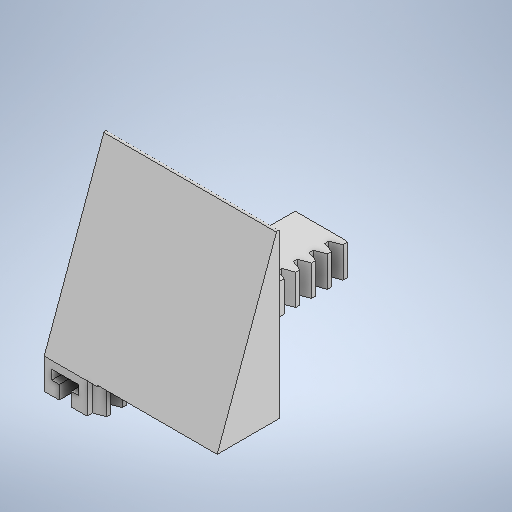
# Autodesk Inventor part: sg90 claw finger
Saved by Autodesk Inventor 2025 (Build 290162000, 162)
## iProperties
Created: 2025-05-11
Part Number: sg90 claw finger
Material: 一般
Document SubType Name: Modeling
Designer: gavin
Density: 1 g/cm^3
Appearance: 預設
Author: gavin
## iProperties of the stored document sg90 claw finger_3D 列印.ipt
Created: 2025-05-11
Part Number: sg90 claw finger_3D 列印
Material: 一般
Document SubType Name: Modeling
Designer: gavin
Density: 1 g/cm^3
Appearance: 預設
Author: gavin
Autodesk Inventor part; units mm, degrees
ref_plane "YZ Plane" through (0, 0, 0) normal (1, 0, 0) x (0, 1, 0)
ref_plane "XZ Plane" through (0, 0, 0) normal (0, 1, 0) x (-1, 0, 0)
sketch "草圖1" plane through (0, 0, 0) normal (0, 0, 1) x (1, 0, 0)
  line L0 (0, -4.2926) -> (-28, -4.2926) projected
  line L1 (0, -4.2926) -> (0, 6.9129) projected
  line L2 (0, 6.9129) -> (1.5, 6.9129) projected
  line L3 (1.5, 6.9129) -> (1.5, 8.4129) projected
  line L4 (1.5, 8.4129) -> (-3.5, 8.4129) projected
  line L5 (-3.5, 8.4129) -> (-3.5, 6.9129) projected
  line L6 (-3.5, 6.9129) -> (-2, 6.9129) projected
  line L7 (-2, 6.9129) -> (-2, 3.81) projected
  line L8 (-2, 3.81) -> (-26, 3.81) projected
  line L9 (-26, 3.81) -> (-26, 6.9129) projected
  line L10 (-26, 6.9129) -> (-24.5, 6.9129) projected
  line L11 (-24.5, 6.9129) -> (-24.5, 8.4129) projected
  line L12 (-24.5, 8.4129) -> (-29.5, 8.4129) projected
  line L13 (-29.5, 8.4129) -> (-29.5, 6.9129) projected
  line L14 (-29.5, 6.9129) -> (-28, 6.9129) projected
  line L15 (-28, -4.2926) -> (-28, 6.9129) projected
  line L16 (-25.8, 4.01) -> (-2.2, 4.01)
  line L17 (-2.2, 4.01) -> (-2.2, 6.7129)
  line L18 (-2.2, 6.7129) -> (-3.7, 6.7129)
  line L19 (-3.7, 6.7129) -> (-3.7, 8.6129)
  line L20 (-3.7, 8.6129) -> (1.7, 8.6129)
  line L21 (1.7, 8.6129) -> (1.7, 6.7129)
  line L22 (1.7, 6.7129) -> (0.2, 6.7129)
  line L23 (0.2, 6.7129) -> (0.2, -4.4926)
  line L24 (0.2, -4.4926) -> (-28.2, -4.4926)
  line L25 (-28.2, -4.4926) -> (-28.2, 6.7129)
  line L26 (-28.2, 6.7129) -> (-29.7, 6.7129)
  line L27 (-29.7, 6.7129) -> (-29.7, 8.6129)
  line L28 (-29.7, 8.6129) -> (-24.3, 8.6129)
  line L29 (-24.3, 8.6129) -> (-24.3, 6.7129)
  line L30 (-24.3, 6.7129) -> (-25.8, 6.7129)
  line L31 (-25.8, 6.7129) -> (-25.8, 4.01)
  line L32 (-23.8, 4.01) -> (-23.8, 10.1129)
  line L33 (-23.8, 10.1129) -> (-31.2, 10.1129)
  line L34 (-31.2, 10.1129) -> (-31.2, 4.01)
  line L35 (-31.2, 4.01) -> (-28.2, 4.01)
  point P0 (0, 0)
  point P1 (-31.2, 7.0615)
  point P2 (-23.8, 7.0615)
  point P3 (-29.7, 4.01)
  dimension "d0" = 0.2
  dimension "d1" = 1.5
  dimension "d2" = 0.5
  dimension "d3" = 1.5
  constraints: 40 end point, 3 midpoint, 3 perpendicular, 2 point on line, 1 horizontal alignment, 1 vertical, 15 other
  measures "d0" distance between parallel lines of L8 L16
  measures "d1" distance from line of point (-31.2, 7.061) L27
  measures "d2" distance from line of point (-23.8, 7.061) L29
  measures "d3" distance between parallel lines of L28 L33
ref_plane "工作平面1" through (-29.5, -4.2926, -50) normal (0, 0, -1) x (0, 1, 0)
extrude "擠出1" add sketch "草圖1" against normal up to surface (50 mm away) contours L31 L30 L29 L28 L27 L26 L25 L35 L34 L33 L32 L16
sketch "草圖2" plane through (-31.2, 10.1129, 0) normal (0, 1, 0) x (1, 0, 0)
  circle A0 centre (17.2, 25) radius 1 projected
  spline S0 degree 3 poles (20.638, 31.1549) (20.6159, 31.1126) (20.5826, 31.049) (20.5316, 30.968) (20.489, 30.9103) (20.4434, 30.8548) (20.393, 30.8037) (20.3395, 30.7558) (20.281, 30.7141) (20.2184, 30.6788) (20.152, 30.6512) (20.0825, 30.6328) (20.011, 30.6244) (19.9391, 30.627) (19.8684, 30.6405) (19.8012, 30.6662) (19.7364, 30.6968) (19.6702, 30.7245) (19.6062, 30.7572) (19.5488, 30.8007) (19.4988, 30.8524) (19.4572, 30.9112) (19.4244, 30.9752) (19.4005, 31.043) (19.3848, 31.1131) (19.3766, 31.1845) (19.3764, 31.2563) (19.3807, 31.328) (19.3915, 31.3989) (19.4058, 31.4693) (19.4319, 31.5613) (19.4569, 31.6286) (19.4735, 31.6734) knots -0.22945 -0.22945 -0.22945 -0.22945 -0.21511 -0.207939 -0.200767 -0.193594 -0.186424 -0.179252 -0.17208 -0.164908 -0.157739 -0.150569 -0.143398 -0.136229 -0.129062 -0.121897 -0.114725 -0.107553 -0.100388 -0.093221 -0.086052 -0.078881 -0.071711 -0.064542 -0.05737 -0.050197 -0.043026 -0.035856 -0.028683 -0.021511 -0.01434 0 0 0 0 projected
  spline S1 degree 3 poles (19.4735, 31.6734) (19.4811, 31.7051) (19.4963, 31.7685) (19.5071, 31.8658) (19.5135, 31.9634) (19.5154, 32.0938) (19.5078, 32.2567) (19.4855, 32.451) (19.4519, 32.6437) (19.4081, 32.8343) (19.3559, 33.0228) (19.3139, 33.1463) (19.293, 33.208) knots -0.156401 -0.156401 -0.156401 -0.156401 -0.146631 -0.136856 -0.127081 -0.117305 -0.097756 -0.078206 -0.058655 -0.039103 -0.019552 0 0 0 0 projected
  arc A1 (19.293, 33.208) -> (18.6265, 33.3497) centre (17.2, 25) ccw projected
  spline S2 degree 3 poles (18.6265, 33.3497) (18.5822, 33.3018) (18.4937, 33.2061) (18.3693, 33.0552) (18.2517, 32.8988) (18.1427, 32.7364) (18.0433, 32.568) (17.9701, 32.4222) (17.9188, 32.3023) (17.8849, 32.2106) (17.8553, 32.1173) (17.8433, 32.0532) (17.8374, 32.0212) knots -0.156401 -0.156401 -0.156401 -0.156401 -0.13685 -0.117298 -0.097746 -0.078195 -0.058645 -0.039096 -0.02932 -0.019545 -0.00977 0 0 0 0 projected
  spline S3 degree 3 poles (17.8374, 32.0212) (17.8343, 31.9735) (17.8298, 31.9019) (17.8162, 31.8071) (17.8007, 31.7371) (17.7816, 31.6679) (17.7564, 31.6007) (17.727, 31.5352) (17.6905, 31.4733) (17.6477, 31.4156) (17.5983, 31.3633) (17.5422, 31.3182) (17.4804, 31.2814) (17.4136, 31.2546) (17.3435, 31.2382) (17.2717, 31.2343) (17.2, 31.2359) (17.1283, 31.2343) (17.0565, 31.2382) (16.9864, 31.2546) (16.9196, 31.2814) (16.8578, 31.3182) (16.8017, 31.3633) (16.7523, 31.4156) (16.7095, 31.4733) (16.673, 31.5352) (16.6436, 31.6007) (16.6184, 31.6679) (16.5993, 31.7371) (16.5838, 31.8071) (16.5702, 31.9019) (16.5657, 31.9735) (16.5626, 32.0212) knots -0.22945 -0.22945 -0.22945 -0.22945 -0.21511 -0.207939 -0.200767 -0.193594 -0.186424 -0.179252 -0.17208 -0.164908 -0.157739 -0.150569 -0.143398 -0.136229 -0.129062 -0.121897 -0.114725 -0.107553 -0.100388 -0.093221 -0.086052 -0.078881 -0.071711 -0.064542 -0.05737 -0.050197 -0.043026 -0.035856 -0.028683 -0.021511 -0.01434 0 0 0 0 projected
  spline S4 degree 3 poles (16.5626, 32.0212) (16.5567, 32.0532) (16.5447, 32.1173) (16.5151, 32.2106) (16.4812, 32.3023) (16.4299, 32.4222) (16.3567, 32.568) (16.2573, 32.7364) (16.1483, 32.8988) (16.0307, 33.0552) (15.9063, 33.2061) (15.8178, 33.3018) (15.7735, 33.3497) knots -0.156401 -0.156401 -0.156401 -0.156401 -0.146631 -0.136856 -0.127081 -0.117305 -0.097756 -0.078206 -0.058655 -0.039103 -0.019552 0 0 0 0 projected
  arc A2 (15.7735, 33.3497) -> (15.107, 33.208) centre (17.2, 25) ccw projected
  spline S5 degree 3 poles (15.107, 33.208) (15.0861, 33.1463) (15.0441, 33.0228) (14.9919, 32.8343) (14.9481, 32.6437) (14.9145, 32.451) (14.8922, 32.2567) (14.8846, 32.0938) (14.8865, 31.9634) (14.8929, 31.8658) (14.9037, 31.7685) (14.9189, 31.7051) (14.9265, 31.6734) knots -0.156401 -0.156401 -0.156401 -0.156401 -0.13685 -0.117298 -0.097746 -0.078195 -0.058645 -0.039096 -0.02932 -0.019545 -0.00977 0 0 0 0 projected
  spline S6 degree 3 poles (14.9265, 31.6734) (14.9431, 31.6286) (14.9681, 31.5613) (14.9942, 31.4693) (15.0085, 31.3989) (15.0193, 31.328) (15.0236, 31.2563) (15.0234, 31.1845) (15.0152, 31.1131) (14.9995, 31.043) (14.9756, 30.9752) (14.9428, 30.9112) (14.9012, 30.8524) (14.8512, 30.8007) (14.7938, 30.7572) (14.7298, 30.7245) (14.6636, 30.6968) (14.5988, 30.6662) (14.5316, 30.6405) (14.4609, 30.627) (14.389, 30.6244) (14.3175, 30.6328) (14.248, 30.6512) (14.1816, 30.6788) (14.119, 30.7141) (14.0605, 30.7558) (14.007, 30.8037) (13.9566, 30.8548) (13.911, 30.9103) (13.8684, 30.968) (13.8174, 31.049) (13.7841, 31.1126) (13.762, 31.1549) knots -0.22945 -0.22945 -0.22945 -0.22945 -0.21511 -0.207939 -0.200767 -0.193594 -0.186424 -0.179252 -0.17208 -0.164908 -0.157739 -0.150569 -0.143398 -0.136229 -0.129062 -0.121897 -0.114725 -0.107553 -0.100388 -0.093221 -0.086052 -0.078881 -0.071711 -0.064542 -0.05737 -0.050197 -0.043026 -0.035856 -0.028683 -0.021511 -0.01434 0 0 0 0 projected
  spline S7 degree 3 poles (13.762, 31.1549) (13.7435, 31.1818) (13.7065, 31.2355) (13.6414, 31.3087) (13.5732, 31.3787) (13.4776, 31.4673) (13.3515, 31.5707) (13.1921, 31.6842) (13.0264, 31.7882) (12.8555, 31.8832) (12.6804, 31.9704) (12.5606, 32.0219) (12.5007, 32.0476) knots -0.156401 -0.156401 -0.156401 -0.156401 -0.146631 -0.136856 -0.127081 -0.117305 -0.097756 -0.078206 -0.058655 -0.039103 -0.019552 0 0 0 0 projected
  arc A3 (12.5007, 32.0476) -> (11.9495, 31.6471) centre (17.2, 25) ccw projected
  spline S8 degree 3 poles (11.9495, 31.6471) (11.9554, 31.5822) (11.9673, 31.4524) (11.9963, 31.2589) (12.0338, 31.0669) (12.0815, 30.8772) (12.1402, 30.6906) (12.1995, 30.5387) (12.2543, 30.4204) (12.2998, 30.3339) (12.3492, 30.2494) (12.3889, 30.1976) (12.4087, 30.1717) knots -0.156401 -0.156401 -0.156401 -0.156401 -0.13685 -0.117298 -0.097746 -0.078195 -0.058645 -0.039096 -0.02932 -0.019545 -0.00977 0 0 0 0 projected
  spline S9 degree 3 poles (12.4087, 30.1717) (12.4422, 30.1376) (12.4923, 30.0863) (12.5536, 30.0128) (12.5953, 29.9544) (12.634, 29.8939) (12.6671, 29.8302) (12.6961, 29.7645) (12.7176, 29.696) (12.7319, 29.6255) (12.7376, 29.5539) (12.7337, 29.482) (12.7196, 29.4115) (12.6949, 29.3439) (12.6601, 29.2808) (12.615, 29.2248) (12.5658, 29.1726) (12.5191, 29.1183) (12.4681, 29.0675) (12.409, 29.0264) (12.3444, 28.9948) (12.2757, 28.9734) (12.2046, 28.9619) (12.1328, 28.9602) (12.0612, 28.9669) (11.9908, 28.9812) (11.9224, 29.0032) (11.8556, 29.0294) (11.7914, 29.0616) (11.729, 29.0969) (11.6495, 29.1502) (11.5933, 29.1947) (11.5558, 29.2244) knots -0.22945 -0.22945 -0.22945 -0.22945 -0.21511 -0.207939 -0.200767 -0.193594 -0.186424 -0.179252 -0.17208 -0.164908 -0.157739 -0.150569 -0.143398 -0.136229 -0.129062 -0.121897 -0.114725 -0.107553 -0.100388 -0.093221 -0.086052 -0.078881 -0.071711 -0.064542 -0.05737 -0.050197 -0.043026 -0.035856 -0.028683 -0.021511 -0.01434 0 0 0 0 projected
  spline S10 degree 3 poles (11.5558, 29.2244) (11.528, 29.2414) (11.4723, 29.2755) (11.3831, 29.3159) (11.2923, 29.3521) (11.1689, 29.3941) (11.0116, 29.4373) (10.8199, 29.4761) (10.6263, 29.5038) (10.4315, 29.521) (10.236, 29.5295) (10.1057, 29.5278) (10.0405, 29.5269) knots -0.156401 -0.156401 -0.156401 -0.156401 -0.146631 -0.136856 -0.127081 -0.117305 -0.097756 -0.078206 -0.058655 -0.039103 -0.019552 0 0 0 0 projected
  arc A4 (10.0405, 29.5269) -> (9.6998, 28.9369) centre (17.2, 25) ccw projected
  spline S11 degree 3 poles (9.6998, 28.9369) (9.7316, 28.88) (9.7953, 28.7662) (9.9004, 28.6012) (10.0128, 28.4411) (10.1335, 28.2872) (10.263, 28.1406) (10.379, 28.026) (10.4772, 27.9402) (10.5539, 27.8796) (10.6335, 27.8226) (10.6908, 27.7914) (10.7194, 27.7758) knots -0.156401 -0.156401 -0.156401 -0.156401 -0.13685 -0.117298 -0.097746 -0.078195 -0.058645 -0.039096 -0.02932 -0.019545 -0.00977 0 0 0 0 projected
  spline S12 degree 3 poles (10.7194, 27.7758) (10.7639, 27.7582) (10.8306, 27.7318) (10.9164, 27.6896) (10.9783, 27.6532) (11.0382, 27.6137) (11.0943, 27.5689) (11.1476, 27.5207) (11.1951, 27.4668) (11.2368, 27.4083) (11.2712, 27.3451) (11.2968, 27.2779) (11.3126, 27.2077) (11.3175, 27.1359) (11.3115, 27.0642) (11.293, 26.9947) (11.2693, 26.927) (11.2487, 26.8583) (11.2228, 26.7912) (11.1855, 26.7296) (11.1394, 26.6744) (11.0853, 26.6269) (11.0251, 26.5876) (10.9601, 26.5568) (10.892, 26.5339) (10.8218, 26.5182) (10.7505, 26.5105) (10.6787, 26.5073) (10.607, 26.5106) (10.5356, 26.5175) (10.4413, 26.5338) (10.3718, 26.5516) (10.3255, 26.5635) knots -0.22945 -0.22945 -0.22945 -0.22945 -0.21511 -0.207939 -0.200767 -0.193594 -0.186424 -0.179252 -0.17208 -0.164908 -0.157739 -0.150569 -0.143398 -0.136229 -0.129062 -0.121897 -0.114725 -0.107553 -0.100388 -0.093221 -0.086052 -0.078881 -0.071711 -0.064542 -0.05737 -0.050197 -0.043026 -0.035856 -0.028683 -0.021511 -0.01434 0 0 0 0 projected
  spline S13 degree 3 poles (10.3255, 26.5635) (10.2932, 26.5677) (10.2285, 26.5762) (10.1306, 26.5768) (10.0329, 26.5729) (9.9031, 26.5612) (9.7419, 26.5366) (9.5509, 26.4941) (9.3628, 26.4406) (9.1778, 26.3771) (8.9958, 26.3054) (8.8774, 26.2508) (8.8182, 26.2235) knots -0.156401 -0.156401 -0.156401 -0.156401 -0.146631 -0.136856 -0.127081 -0.117305 -0.097756 -0.078206 -0.058655 -0.039103 -0.019552 0 0 0 0 projected
  arc A5 (8.8182, 26.2235) -> (8.747, 25.5459) centre (17.2, 25) ccw projected
  spline S14 degree 3 poles (8.747, 25.5459) (8.7992, 25.5069) (8.9036, 25.4288) (9.0667, 25.3209) (9.2345, 25.2203) (9.4074, 25.1289) (9.5854, 25.0476) (9.7379, 24.9901) (9.8625, 24.9516) (9.9573, 24.9275) (10.0532, 24.9077) (10.1182, 24.9025) (10.1507, 24.9) knots -0.156401 -0.156401 -0.156401 -0.156401 -0.13685 -0.117298 -0.097746 -0.078195 -0.058645 -0.039096 -0.02932 -0.019545 -0.00977 0 0 0 0 projected
  spline S15 degree 3 poles (10.1507, 24.9) (10.1984, 24.9019) (10.2701, 24.9049) (10.3657, 24.9013) (10.437, 24.8932) (10.5079, 24.8815) (10.5773, 24.8634) (10.6456, 24.841) (10.7109, 24.8112) (10.7728, 24.7746) (10.8299, 24.7309) (10.8806, 24.6799) (10.9237, 24.6222) (10.9573, 24.5587) (10.981, 24.4906) (10.9924, 24.4196) (10.9982, 24.3482) (11.0073, 24.2771) (11.011, 24.2052) (11.002, 24.1338) (10.9823, 24.0646) (10.9522, 23.9992) (10.9132, 23.9388) (10.8664, 23.8842) (10.8135, 23.8356) (10.7557, 23.7928) (10.6937, 23.7567) (10.6295, 23.7246) (10.5626, 23.6984) (10.4946, 23.6756) (10.4018, 23.6522) (10.3311, 23.6402) (10.2839, 23.6322) knots -0.22945 -0.22945 -0.22945 -0.22945 -0.21511 -0.207939 -0.200767 -0.193594 -0.186424 -0.179252 -0.17208 -0.164908 -0.157739 -0.150569 -0.143398 -0.136229 -0.129062 -0.121897 -0.114725 -0.107553 -0.100388 -0.093221 -0.086052 -0.078881 -0.071711 -0.064542 -0.05737 -0.050197 -0.043026 -0.035856 -0.028683 -0.021511 -0.01434 0 0 0 0 projected
  spline S16 degree 3 poles (10.2839, 23.6322) (10.2527, 23.6229) (10.1901, 23.6044) (10.1005, 23.5651) (10.0128, 23.5218) (9.8989, 23.4583) (9.7617, 23.3703) (9.6045, 23.2538) (9.4544, 23.1284) (9.3112, 22.9951) (9.1741, 22.8556) (9.0882, 22.7576) (9.0452, 22.7086) knots -0.156401 -0.156401 -0.156401 -0.156401 -0.146631 -0.136856 -0.127081 -0.117305 -0.097756 -0.078206 -0.058655 -0.039103 -0.019552 0 0 0 0 projected
  arc A6 (9.0452, 22.7086) -> (9.2557, 22.0605) centre (17.2, 25) ccw projected
  spline S17 degree 3 poles (9.2557, 22.0605) (9.3193, 22.0461) (9.4465, 22.0173) (9.6394, 21.985) (9.8335, 21.9614) (10.0287, 21.9482) (10.2243, 21.9463) (10.3871, 21.9558) (10.5166, 21.9713) (10.6129, 21.9879) (10.7086, 22.0088) (10.7701, 22.0305) (10.8008, 22.0414) knots -0.156401 -0.156401 -0.156401 -0.156401 -0.13685 -0.117298 -0.097746 -0.078195 -0.058645 -0.039096 -0.02932 -0.019545 -0.00977 0 0 0 0 projected
  spline S18 degree 3 poles (10.8008, 22.0414) (10.8436, 22.0626) (10.9079, 22.0945) (10.9967, 22.1301) (11.0652, 22.1517) (11.1346, 22.1698) (11.2055, 22.1815) (11.2769, 22.1888) (11.3488, 22.1881) (11.4201, 22.1799) (11.4901, 22.1632) (11.5572, 22.1373) (11.6199, 22.1021) (11.6766, 22.0577) (11.7258, 22.0052) (11.7651, 21.9449) (11.7995, 21.882) (11.8368, 21.8208) (11.8693, 21.7567) (11.8902, 21.6877) (11.9003, 21.6165) (11.8994, 21.5445) (11.8883, 21.4734) (11.8678, 21.4045) (11.8392, 21.3386) (11.8039, 21.276) (11.7619, 21.2178) (11.7163, 21.1624) (11.6659, 21.1113) (11.6129, 21.0628) (11.5377, 21.0036) (11.478, 20.9639) (11.4382, 20.9374) knots -0.22945 -0.22945 -0.22945 -0.22945 -0.21511 -0.207939 -0.200767 -0.193594 -0.186424 -0.179252 -0.17208 -0.164908 -0.157739 -0.150569 -0.143398 -0.136229 -0.129062 -0.121897 -0.114725 -0.107553 -0.100388 -0.093221 -0.086052 -0.078881 -0.071711 -0.064542 -0.05737 -0.050197 -0.043026 -0.035856 -0.028683 -0.021511 -0.01434 0 0 0 0 projected
  spline S19 degree 3 poles (11.4382, 20.9374) (11.4134, 20.9162) (11.3638, 20.8739) (11.2979, 20.8015) (11.2354, 20.7263) (11.1572, 20.622) (11.0676, 20.4857) (10.9714, 20.3154) (10.8853, 20.1397) (10.8087, 19.9598) (10.7402, 19.7766) (10.7015, 19.6521) (10.6822, 19.5898) knots -0.156401 -0.156401 -0.156401 -0.156401 -0.146631 -0.136856 -0.127081 -0.117305 -0.097756 -0.078206 -0.058655 -0.039103 -0.019552 0 0 0 0 projected
  arc A7 (10.6822, 19.5898) -> (11.1381, 19.0834) centre (17.2, 25) ccw projected
  spline S20 degree 3 poles (11.1381, 19.0834) (11.2021, 19.0961) (11.3299, 19.1215) (11.5193, 19.1705) (11.7063, 19.2279) (11.89, 19.2952) (12.0694, 19.3731) (12.2143, 19.448) (12.3263, 19.5148) (12.4076, 19.5691) (12.4864, 19.6271) (12.5338, 19.672) (12.5574, 19.6944) knots -0.156401 -0.156401 -0.156401 -0.156401 -0.13685 -0.117298 -0.097746 -0.078195 -0.058645 -0.039096 -0.02932 -0.019545 -0.00977 0 0 0 0 projected
  spline S21 degree 3 poles (12.5574, 19.6944) (12.5879, 19.7312) (12.6337, 19.7865) (12.7003, 19.8551) (12.7541, 19.9027) (12.8102, 19.9475) (12.8701, 19.987) (12.9324, 20.0227) (12.9983, 20.0513) (13.0669, 20.0728) (13.1375, 20.0861) (13.2094, 20.0896) (13.281, 20.083) (13.3508, 20.0655) (13.4172, 20.0375) (13.4776, 19.9985) (13.5346, 19.955) (13.5936, 19.9142) (13.6494, 19.8689) (13.6965, 19.8144) (13.7347, 19.7534) (13.7631, 19.6873) (13.7819, 19.6179) (13.7912, 19.5466) (13.7919, 19.4747) (13.7851, 19.4032) (13.7704, 19.3329) (13.7513, 19.2637) (13.726, 19.1965) (13.6974, 19.1307) (13.6527, 19.0461) (13.6143, 18.9855) (13.5887, 18.9451) knots -0.22945 -0.22945 -0.22945 -0.22945 -0.21511 -0.207939 -0.200767 -0.193594 -0.186424 -0.179252 -0.17208 -0.164908 -0.157739 -0.150569 -0.143398 -0.136229 -0.129062 -0.121897 -0.114725 -0.107553 -0.100388 -0.093221 -0.086052 -0.078881 -0.071711 -0.064542 -0.05737 -0.050197 -0.043026 -0.035856 -0.028683 -0.021511 -0.01434 0 0 0 0 projected
  spline S22 degree 3 poles (13.5887, 18.9451) (13.5747, 18.9157) (13.5466, 18.8568) (13.5158, 18.7639) (13.4893, 18.6698) (13.4604, 18.5426) (13.4339, 18.3817) (13.4153, 18.187) (13.4081, 17.9915) (13.4113, 17.796) (13.4232, 17.6007) (13.4386, 17.4712) (13.4462, 17.4065) knots -0.156401 -0.156401 -0.156401 -0.156401 -0.146631 -0.136856 -0.127081 -0.117305 -0.097756 -0.078206 -0.058655 -0.039103 -0.019552 0 0 0 0 projected
  arc A8 (13.4462, 17.4065) -> (14.0687, 17.1294) centre (17.2, 25) ccw projected
  spline S23 degree 3 poles (14.0687, 17.1294) (14.1219, 17.167) (14.2284, 17.2422) (14.3815, 17.364) (14.529, 17.4924) (14.6694, 17.6286) (14.8017, 17.7728) (14.9036, 17.9001) (14.9787, 18.0067) (15.0309, 18.0893) (15.0793, 18.1744) (15.1043, 18.2347) (15.1168, 18.2648) knots -0.156401 -0.156401 -0.156401 -0.156401 -0.13685 -0.117298 -0.097746 -0.078195 -0.058645 -0.039096 -0.02932 -0.019545 -0.00977 0 0 0 0 projected
  spline S24 degree 3 poles (15.1168, 18.2648) (15.1297, 18.3108) (15.149, 18.3799) (15.182, 18.4697) (15.2117, 18.535) (15.2447, 18.5988) (15.2834, 18.6593) (15.3258, 18.7172) (15.3744, 18.7702) (15.4282, 18.8177) (15.4874, 18.8585) (15.5516, 18.891) (15.6198, 18.9141) (15.6907, 18.9265) (15.7627, 18.928) (15.8337, 18.9168) (15.9035, 18.9003) (15.9739, 18.887) (16.0434, 18.8683) (16.1085, 18.8377) (16.1683, 18.7975) (16.2211, 18.7487) (16.2666, 18.6929) (16.304, 18.6316) (16.3339, 18.5662) (16.3568, 18.4981) (16.3719, 18.4279) (16.3826, 18.3569) (16.3868, 18.2853) (16.3875, 18.2135) (16.3811, 18.118) (16.3706, 18.047) (16.3637, 17.9997) knots -0.22945 -0.22945 -0.22945 -0.22945 -0.21511 -0.207939 -0.200767 -0.193594 -0.186424 -0.179252 -0.17208 -0.164908 -0.157739 -0.150569 -0.143398 -0.136229 -0.129062 -0.121897 -0.114725 -0.107553 -0.100388 -0.093221 -0.086052 -0.078881 -0.071711 -0.064542 -0.05737 -0.050197 -0.043026 -0.035856 -0.028683 -0.021511 -0.01434 0 0 0 0 projected
  spline S25 degree 3 poles (16.3637, 17.9997) (16.3628, 17.9671) (16.3612, 17.902) (16.3708, 17.8045) (16.3848, 17.7078) (16.4101, 17.5799) (16.4514, 17.4221) (16.5136, 17.2366) (16.5865, 17.0551) (16.669, 16.8778) (16.7593, 16.7042) (16.826, 16.5922) (16.8593, 16.5362) knots -0.156401 -0.156401 -0.156401 -0.156401 -0.146631 -0.136856 -0.127081 -0.117305 -0.097756 -0.078206 -0.058655 -0.039103 -0.019552 0 0 0 0 projected
  arc A9 (16.8593, 16.5362) -> (17.5407, 16.5362) centre (17.2, 25) ccw projected
  spline S26 degree 3 poles (17.5407, 16.5362) (17.574, 16.5922) (17.6407, 16.7042) (17.731, 16.8778) (17.8135, 17.0551) (17.8864, 17.2366) (17.9486, 17.4221) (17.9899, 17.5799) (18.0152, 17.7078) (18.0292, 17.8045) (18.0388, 17.902) (18.0372, 17.9671) (18.0363, 17.9997) knots -0.156401 -0.156401 -0.156401 -0.156401 -0.13685 -0.117298 -0.097746 -0.078195 -0.058645 -0.039096 -0.02932 -0.019545 -0.00977 0 0 0 0 projected
  spline S27 degree 3 poles (18.0363, 17.9997) (18.0294, 18.047) (18.0189, 18.118) (18.0125, 18.2135) (18.0132, 18.2853) (18.0174, 18.3569) (18.0281, 18.4279) (18.0432, 18.4981) (18.0661, 18.5662) (18.096, 18.6316) (18.1334, 18.6929) (18.1789, 18.7487) (18.2317, 18.7975) (18.2915, 18.8377) (18.3566, 18.8683) (18.4261, 18.887) (18.4965, 18.9003) (18.5663, 18.9168) (18.6373, 18.928) (18.7093, 18.9265) (18.7802, 18.9141) (18.8484, 18.891) (18.9126, 18.8585) (18.9718, 18.8177) (19.0256, 18.7702) (19.0742, 18.7172) (19.1166, 18.6593) (19.1553, 18.5988) (19.1883, 18.535) (19.218, 18.4697) (19.251, 18.3799) (19.2703, 18.3108) (19.2832, 18.2648) knots -0.22945 -0.22945 -0.22945 -0.22945 -0.21511 -0.207939 -0.200767 -0.193594 -0.186424 -0.179252 -0.17208 -0.164908 -0.157739 -0.150569 -0.143398 -0.136229 -0.129062 -0.121897 -0.114725 -0.107553 -0.100388 -0.093221 -0.086052 -0.078881 -0.071711 -0.064542 -0.05737 -0.050197 -0.043026 -0.035856 -0.028683 -0.021511 -0.01434 0 0 0 0 projected
  spline S28 degree 3 poles (19.2832, 18.2648) (19.2957, 18.2347) (19.3207, 18.1744) (19.3691, 18.0893) (19.4213, 18.0067) (19.4964, 17.9001) (19.5983, 17.7728) (19.7306, 17.6286) (19.871, 17.4924) (20.0185, 17.364) (20.1716, 17.2422) (20.2781, 17.167) (20.3313, 17.1294) knots -0.156401 -0.156401 -0.156401 -0.156401 -0.146631 -0.136856 -0.127081 -0.117305 -0.097756 -0.078206 -0.058655 -0.039103 -0.019552 0 0 0 0 projected
  arc A10 (20.3313, 17.1294) -> (20.9538, 17.4065) centre (17.2, 25) ccw projected
  spline S29 degree 3 poles (20.9538, 17.4065) (20.9614, 17.4712) (20.9768, 17.6007) (20.9887, 17.796) (20.9919, 17.9915) (20.9847, 18.187) (20.9661, 18.3817) (20.9396, 18.5426) (20.9107, 18.6698) (20.8842, 18.7639) (20.8534, 18.8568) (20.8253, 18.9157) (20.8113, 18.9451) knots -0.156401 -0.156401 -0.156401 -0.156401 -0.13685 -0.117298 -0.097746 -0.078195 -0.058645 -0.039096 -0.02932 -0.019545 -0.00977 0 0 0 0 projected
  spline S30 degree 3 poles (20.8113, 18.9451) (20.7857, 18.9855) (20.7473, 19.0461) (20.7026, 19.1307) (20.674, 19.1965) (20.6487, 19.2637) (20.6296, 19.3329) (20.6149, 19.4032) (20.6081, 19.4747) (20.6088, 19.5466) (20.6181, 19.6179) (20.6369, 19.6873) (20.6653, 19.7534) (20.7035, 19.8144) (20.7506, 19.8689) (20.8064, 19.9142) (20.8654, 19.955) (20.9224, 19.9985) (20.9828, 20.0375) (21.0492, 20.0655) (21.119, 20.083) (21.1906, 20.0896) (21.2625, 20.0861) (21.3331, 20.0728) (21.4017, 20.0513) (21.4676, 20.0227) (21.5299, 19.987) (21.5898, 19.9475) (21.6459, 19.9027) (21.6997, 19.8551) (21.7663, 19.7865) (21.8121, 19.7312) (21.8426, 19.6944) knots -0.22945 -0.22945 -0.22945 -0.22945 -0.21511 -0.207939 -0.200767 -0.193594 -0.186424 -0.179252 -0.17208 -0.164908 -0.157739 -0.150569 -0.143398 -0.136229 -0.129062 -0.121897 -0.114725 -0.107553 -0.100388 -0.093221 -0.086052 -0.078881 -0.071711 -0.064542 -0.05737 -0.050197 -0.043026 -0.035856 -0.028683 -0.021511 -0.01434 0 0 0 0 projected
  spline S31 degree 3 poles (21.8426, 19.6944) (21.8662, 19.672) (21.9136, 19.6271) (21.9924, 19.5691) (22.0737, 19.5148) (22.1857, 19.448) (22.3306, 19.3731) (22.51, 19.2952) (22.6937, 19.2279) (22.8807, 19.1705) (23.0701, 19.1215) (23.1979, 19.0961) (23.2619, 19.0834) knots -0.156401 -0.156401 -0.156401 -0.156401 -0.146631 -0.136856 -0.127081 -0.117305 -0.097756 -0.078206 -0.058655 -0.039103 -0.019552 0 0 0 0 projected
  arc A11 (23.2619, 19.0834) -> (23.7178, 19.5898) centre (17.2, 25) ccw projected
  spline S32 degree 3 poles (23.7178, 19.5898) (23.6985, 19.6521) (23.6598, 19.7766) (23.5913, 19.9598) (23.5147, 20.1397) (23.4286, 20.3154) (23.3324, 20.4857) (23.2428, 20.622) (23.1646, 20.7263) (23.1021, 20.8015) (23.0362, 20.8739) (22.9866, 20.9162) (22.9618, 20.9374) knots -0.156401 -0.156401 -0.156401 -0.156401 -0.13685 -0.117298 -0.097746 -0.078195 -0.058645 -0.039096 -0.02932 -0.019545 -0.00977 0 0 0 0 projected
  spline S33 degree 3 poles (22.9618, 20.9374) (22.922, 20.9639) (22.8623, 21.0036) (22.7871, 21.0628) (22.7341, 21.1113) (22.6837, 21.1624) (22.6381, 21.2178) (22.5961, 21.276) (22.5608, 21.3386) (22.5322, 21.4045) (22.5117, 21.4734) (22.5006, 21.5445) (22.4997, 21.6165) (22.5098, 21.6877) (22.5307, 21.7567) (22.5632, 21.8208) (22.6005, 21.882) (22.6349, 21.9449) (22.6742, 22.0052) (22.7234, 22.0577) (22.7801, 22.1021) (22.8428, 22.1373) (22.9099, 22.1632) (22.9799, 22.1799) (23.0512, 22.1881) (23.1231, 22.1888) (23.1945, 22.1815) (23.2654, 22.1698) (23.3348, 22.1517) (23.4033, 22.1301) (23.4921, 22.0945) (23.5564, 22.0626) (23.5992, 22.0414) knots -0.22945 -0.22945 -0.22945 -0.22945 -0.21511 -0.207939 -0.200767 -0.193594 -0.186424 -0.179252 -0.17208 -0.164908 -0.157739 -0.150569 -0.143398 -0.136229 -0.129062 -0.121897 -0.114725 -0.107553 -0.100388 -0.093221 -0.086052 -0.078881 -0.071711 -0.064542 -0.05737 -0.050197 -0.043026 -0.035856 -0.028683 -0.021511 -0.01434 0 0 0 0 projected
  spline S34 degree 3 poles (23.5992, 22.0414) (23.6299, 22.0305) (23.6914, 22.0088) (23.7871, 21.9879) (23.8834, 21.9713) (24.0129, 21.9558) (24.1757, 21.9463) (24.3713, 21.9482) (24.5665, 21.9614) (24.7606, 21.985) (24.9535, 22.0173) (25.0807, 22.0461) (25.1443, 22.0605) knots -0.156401 -0.156401 -0.156401 -0.156401 -0.146631 -0.136856 -0.127081 -0.117305 -0.097756 -0.078206 -0.058655 -0.039103 -0.019552 0 0 0 0 projected
  arc A12 (25.1443, 22.0605) -> (25.3548, 22.7086) centre (17.2, 25) ccw projected
  spline S35 degree 3 poles (25.3548, 22.7086) (25.3118, 22.7576) (25.2259, 22.8556) (25.0888, 22.9951) (24.9456, 23.1284) (24.7955, 23.2538) (24.6383, 23.3703) (24.5011, 23.4583) (24.3872, 23.5218) (24.2995, 23.5651) (24.2099, 23.6044) (24.1473, 23.6229) (24.1161, 23.6322) knots -0.156401 -0.156401 -0.156401 -0.156401 -0.13685 -0.117298 -0.097746 -0.078195 -0.058645 -0.039096 -0.02932 -0.019545 -0.00977 0 0 0 0 projected
  spline S36 degree 3 poles (24.1161, 23.6322) (24.0689, 23.6402) (23.9982, 23.6522) (23.9054, 23.6756) (23.8374, 23.6984) (23.7705, 23.7246) (23.7063, 23.7567) (23.6443, 23.7928) (23.5865, 23.8356) (23.5336, 23.8842) (23.4868, 23.9388) (23.4478, 23.9992) (23.4177, 24.0646) (23.398, 24.1338) (23.389, 24.2052) (23.3927, 24.2771) (23.4018, 24.3482) (23.4076, 24.4196) (23.419, 24.4906) (23.4427, 24.5587) (23.4763, 24.6222) (23.5194, 24.6799) (23.5701, 24.7309) (23.6272, 24.7746) (23.6891, 24.8112) (23.7544, 24.841) (23.8227, 24.8634) (23.8921, 24.8815) (23.963, 24.8932) (24.0343, 24.9013) (24.1299, 24.9049) (24.2016, 24.9019) (24.2493, 24.9) knots -0.22945 -0.22945 -0.22945 -0.22945 -0.21511 -0.207939 -0.200767 -0.193594 -0.186424 -0.179252 -0.17208 -0.164908 -0.157739 -0.150569 -0.143398 -0.136229 -0.129062 -0.121897 -0.114725 -0.107553 -0.100388 -0.093221 -0.086052 -0.078881 -0.071711 -0.064542 -0.05737 -0.050197 -0.043026 -0.035856 -0.028683 -0.021511 -0.01434 0 0 0 0 projected
  spline S37 degree 3 poles (24.2493, 24.9) (24.2818, 24.9025) (24.3468, 24.9077) (24.4427, 24.9275) (24.5375, 24.9516) (24.6621, 24.9901) (24.8146, 25.0476) (24.9926, 25.1289) (25.1655, 25.2203) (25.3333, 25.3209) (25.4964, 25.4288) (25.6008, 25.5069) (25.653, 25.5459) knots -0.156401 -0.156401 -0.156401 -0.156401 -0.146631 -0.136856 -0.127081 -0.117305 -0.097756 -0.078206 -0.058655 -0.039103 -0.019552 0 0 0 0 projected
  arc A13 (25.653, 25.5459) -> (25.5818, 26.2235) centre (17.2, 25) ccw projected
  spline S38 degree 3 poles (25.5818, 26.2235) (25.5226, 26.2508) (25.4042, 26.3054) (25.2222, 26.3771) (25.0372, 26.4406) (24.8491, 26.4941) (24.6581, 26.5366) (24.4969, 26.5612) (24.3671, 26.5729) (24.2694, 26.5768) (24.1715, 26.5762) (24.1068, 26.5677) (24.0745, 26.5635) knots -0.156401 -0.156401 -0.156401 -0.156401 -0.13685 -0.117298 -0.097746 -0.078195 -0.058645 -0.039096 -0.02932 -0.019545 -0.00977 0 0 0 0 projected
  spline S39 degree 3 poles (24.0745, 26.5635) (24.0282, 26.5516) (23.9587, 26.5338) (23.8644, 26.5175) (23.793, 26.5106) (23.7213, 26.5073) (23.6495, 26.5105) (23.5782, 26.5182) (23.508, 26.5339) (23.4399, 26.5568) (23.3749, 26.5876) (23.3147, 26.6269) (23.2606, 26.6744) (23.2145, 26.7296) (23.1772, 26.7912) (23.1513, 26.8583) (23.1307, 26.927) (23.107, 26.9947) (23.0885, 27.0642) (23.0825, 27.1359) (23.0874, 27.2077) (23.1032, 27.2779) (23.1288, 27.3451) (23.1632, 27.4083) (23.2049, 27.4668) (23.2524, 27.5207) (23.3057, 27.5689) (23.3618, 27.6137) (23.4217, 27.6532) (23.4836, 27.6896) (23.5694, 27.7318) (23.6361, 27.7582) (23.6806, 27.7758) knots -0.22945 -0.22945 -0.22945 -0.22945 -0.21511 -0.207939 -0.200767 -0.193594 -0.186424 -0.179252 -0.17208 -0.164908 -0.157739 -0.150569 -0.143398 -0.136229 -0.129062 -0.121897 -0.114725 -0.107553 -0.100388 -0.093221 -0.086052 -0.078881 -0.071711 -0.064542 -0.05737 -0.050197 -0.043026 -0.035856 -0.028683 -0.021511 -0.01434 0 0 0 0 projected
  spline S40 degree 3 poles (23.6806, 27.7758) (23.7092, 27.7914) (23.7665, 27.8226) (23.8461, 27.8796) (23.9228, 27.9402) (24.021, 28.026) (24.137, 28.1406) (24.2665, 28.2872) (24.3872, 28.4411) (24.4996, 28.6012) (24.6047, 28.7662) (24.6684, 28.88) (24.7002, 28.9369) knots -0.156401 -0.156401 -0.156401 -0.156401 -0.146631 -0.136856 -0.127081 -0.117305 -0.097756 -0.078206 -0.058655 -0.039103 -0.019552 0 0 0 0 projected
  arc A14 (24.7002, 28.9369) -> (24.3595, 29.5269) centre (17.2, 25) ccw projected
  spline S41 degree 3 poles (24.3595, 29.5269) (24.2943, 29.5278) (24.164, 29.5295) (23.9685, 29.521) (23.7737, 29.5038) (23.5801, 29.4761) (23.3884, 29.4373) (23.2311, 29.3941) (23.1077, 29.3521) (23.0169, 29.3159) (22.9277, 29.2755) (22.872, 29.2414) (22.8442, 29.2244) knots -0.156401 -0.156401 -0.156401 -0.156401 -0.13685 -0.117298 -0.097746 -0.078195 -0.058645 -0.039096 -0.02932 -0.019545 -0.00977 0 0 0 0 projected
  spline S42 degree 3 poles (22.8442, 29.2244) (22.8067, 29.1947) (22.7505, 29.1502) (22.671, 29.0969) (22.6086, 29.0616) (22.5444, 29.0294) (22.4776, 29.0032) (22.4092, 28.9812) (22.3388, 28.9669) (22.2672, 28.9602) (22.1954, 28.9619) (22.1243, 28.9734) (22.0556, 28.9948) (21.991, 29.0264) (21.9319, 29.0675) (21.8809, 29.1183) (21.8342, 29.1726) (21.785, 29.2248) (21.7399, 29.2808) (21.7051, 29.3439) (21.6804, 29.4115) (21.6663, 29.482) (21.6624, 29.5539) (21.6681, 29.6255) (21.6824, 29.696) (21.7039, 29.7645) (21.7329, 29.8302) (21.766, 29.8939) (21.8047, 29.9544) (21.8464, 30.0128) (21.9077, 30.0863) (21.9578, 30.1376) (21.9913, 30.1717) knots -0.22945 -0.22945 -0.22945 -0.22945 -0.21511 -0.207939 -0.200767 -0.193594 -0.186424 -0.179252 -0.17208 -0.164908 -0.157739 -0.150569 -0.143398 -0.136229 -0.129062 -0.121897 -0.114725 -0.107553 -0.100388 -0.093221 -0.086052 -0.078881 -0.071711 -0.064542 -0.05737 -0.050197 -0.043026 -0.035856 -0.028683 -0.021511 -0.01434 0 0 0 0 projected
  spline S43 degree 3 poles (21.9913, 30.1717) (22.0111, 30.1976) (22.0508, 30.2494) (22.1002, 30.3339) (22.1457, 30.4204) (22.2005, 30.5387) (22.2598, 30.6906) (22.3185, 30.8772) (22.3662, 31.0669) (22.4037, 31.2589) (22.4327, 31.4524) (22.4446, 31.5822) (22.4505, 31.6471) knots -0.156401 -0.156401 -0.156401 -0.156401 -0.146631 -0.136856 -0.127081 -0.117305 -0.097756 -0.078206 -0.058655 -0.039103 -0.019552 0 0 0 0 projected
  arc A15 (22.4505, 31.6471) -> (21.8993, 32.0476) centre (17.2, 25) ccw projected
  spline S44 degree 3 poles (21.8993, 32.0476) (21.8394, 32.0219) (21.7196, 31.9704) (21.5445, 31.8832) (21.3736, 31.7882) (21.2079, 31.6842) (21.0485, 31.5707) (20.9224, 31.4673) (20.8268, 31.3787) (20.7586, 31.3087) (20.6935, 31.2355) (20.6565, 31.1818) (20.638, 31.1549) knots -0.156401 -0.156401 -0.156401 -0.156401 -0.13685 -0.117298 -0.097746 -0.078195 -0.058645 -0.039096 -0.02932 -0.019545 -0.00977 0 0 0 0 projected
  line L0 (8.5297, 16.7951) -> (10.5797, 17.5412)
  line L1 (10.5797, 17.5412) -> (10.5797, 18.3841)
  line L2 (10.5797, 18.3841) -> (8.5297, 19.1302)
  line L3 (8.5297, 19.1302) -> (8.5297, 19.9367)
  line L4 (8.5297, 19.9367) -> (10.5797, 20.6828)
  line L5 (10.5797, 20.6828) -> (10.5797, 21.5257)
  line L6 (10.5797, 21.5257) -> (8.5297, 22.2718)
  line L7 (8.5297, 22.2718) -> (8.5297, 23.0783)
  line L8 (8.5297, 23.0783) -> (10.5797, 23.8244)
  line L9 (10.5797, 23.8244) -> (10.5797, 24.6673)
  line L10 (10.5797, 24.6673) -> (8.5297, 25.4134)
  line L11 (8.5297, 25.4134) -> (8.5297, 26.2199)
  line L12 (8.5297, 26.2199) -> (10.5797, 26.966)
  line L13 (10.5797, 26.966) -> (10.5797, 27.8089)
  line L14 (10.5797, 27.8089) -> (8.5297, 28.555)
  line L15 (8.5297, 28.555) -> (8.5297, 29.3615)
  line L16 (8.5297, 29.3615) -> (10.5797, 30.1076)
  line L17 (10.5797, 30.1076) -> (10.5797, 30.9504)
  line L18 (10.5797, 30.9504) -> (8.5297, 31.6966)
  line L19 (7.4, 0) -> (7.4, 50) projected
  line L20 (8.5297, 13.6535) -> (10.5797, 14.3996)
  line L21 (10.5797, 14.3996) -> (10.5797, 15.2425)
  line L22 (10.5797, 15.2425) -> (8.5297, 15.9886)
  line L23 (8.5297, 15.9886) -> (8.5297, 16.7951)
  line L24 (8.5297, 10.5119) -> (10.5797, 11.258)
  line L25 (10.5797, 11.258) -> (10.5797, 12.1009)
  line L26 (10.5797, 12.1009) -> (8.5297, 12.847)
  line L27 (8.5297, 12.847) -> (8.5297, 13.6535)
  line L28 (8.5297, 7.3703) -> (10.5797, 8.1164)
  line L29 (10.5797, 8.1164) -> (10.5797, 8.9593)
  line L30 (10.5797, 8.9593) -> (8.5297, 9.7054)
  line L31 (8.5297, 9.7054) -> (8.5297, 10.5119)
  line L32 (8.5297, 4.2287) -> (10.5797, 4.9748)
  line L33 (10.5797, 4.9748) -> (10.5797, 5.8177)
  line L34 (10.5797, 5.8177) -> (8.5297, 6.5638)
  line L35 (8.5297, 6.5638) -> (8.5297, 7.3703)
  line L36 (8.5297, 1.0871) -> (10.5797, 1.8333)
  line L37 (10.5797, 1.8333) -> (10.5797, 2.6761)
  line L38 (10.5797, 2.6761) -> (8.5297, 3.4223)
  line L39 (8.5297, 3.4223) -> (8.5297, 4.2287)
  line L40 (8.5297, 31.6966) -> (8.5297, 32.503)
  line L41 (8.5297, 32.503) -> (10.5797, 33.2492)
  line L42 (10.5797, 33.2492) -> (10.5797, 34.092)
  line L43 (10.5797, 34.092) -> (8.5297, 34.8382)
  line L44 (8.5297, 34.8382) -> (8.5297, 35.6446)
  line L45 (8.5297, 35.6446) -> (10.5797, 36.3908)
  line L46 (10.5797, 36.3908) -> (10.5797, 37.2336)
  line L47 (10.5797, 37.2336) -> (8.5297, 37.9798)
  line L48 (8.5297, 37.9798) -> (8.5297, 38.7862)
  line L49 (8.5297, 38.7862) -> (10.5797, 39.5324)
  line L50 (10.5797, 39.5324) -> (10.5797, 40.3752)
  line L51 (10.5797, 40.3752) -> (8.5297, 41.1214)
  line L52 (8.5297, 41.1214) -> (8.5297, 41.9278)
  line L53 (8.5297, 41.9278) -> (10.5797, 42.674)
  line L54 (10.5797, 42.674) -> (10.5797, 43.5168)
  line L55 (10.5797, 43.5168) -> (8.5297, 44.263)
  line L56 (8.5297, 44.263) -> (8.5297, 45.0694)
  line L57 (8.5297, 45.0694) -> (10.5797, 45.8156)
  line L58 (10.5797, 45.8156) -> (10.5797, 46.6584)
  line L59 (10.5797, 46.6584) -> (8.5297, 47.4045)
  line L60 (8.5297, 47.4045) -> (8.5297, 48.211)
  line L61 (8.5297, 48.211) -> (10.5797, 48.9571)
  line L62 (10.5797, 48.9571) -> (10.5797, 49.8)
  line L63 (10.5797, 49.8) -> (8.5297, 50.5461)
  line L64 (7.4, 50) -> (10.0302, 50)
  line L65 (8.5297, 0.2807) -> (8.5297, 1.0871)
  line L66 (8.5297, 0.2807) -> (8.5297, 0)
  line L67 (8.5297, 0) -> (7.4, 0)
  point P0 (31.2, 0)
  constraints: 134 end point, 1 horizontal, 1 perpendicular, 1 point on line, 1 vertical
extrude "擠出2" add sketch "草圖2" against normal up to surface (6.1029 mm away) contours L23 L22 L21 L20 L27 L26 L25 L24 L31 L30 L29 L28 L35 L34 L33 L32 L39 L38 L37 L36 L65 L66 L67 L19 L64 L63 L62 L61 L60 L59 L58 L57 L56 L55 L54 L53 L52 L51 L50 L49 L48 L47 L46 L45 L44 L43 L42 L41 L40 L18 L17 L16 L15 L14 L13 L12 L11 L10 L9 L8 L7 L6 L5 L4 L3 L2 L1 L0
sketch "草圖3" plane through (-31.2, 4.01, 0) normal (-1, 0, 0) x (0, 0, 1)
  line L0 (-50, 6.1029) -> (-50, 0) projected
  line L1 (0, 0) -> (-50, 0) projected
  line L2 (0, 6.1029) -> (0, 0) projected
  line L3 (0, 6.1029) -> (-50, 6.1029) projected
  line L4 (0, 6.1029) -> (-5.4596, 21.1029)
  line L5 (-5.4596, 21.1029) -> (-12.4596, 21.1029)
  line L6 (-12.4596, 21.1029) -> (-12.4596, 6.1029)
  point P0 (0, -4.01)
  dimension "d8" = 70
  dimension "d9" = 15
  dimension "d10" = 7
  constraints: 6 end point, 1 horizontal, 1 perpendicular, 1 point on line
  measures "d8" angle of L3 L4
  measures "d9" distance of L5.end L6.end
  measures "d10" distance of L4.end L5.end
extrude "擠出3" add sketch "草圖3" against normal blind 33.4 contours L6 L5 L4 L3
sketch "草圖4" plane through (-31.2, 10.1129, -12.4596) normal (0, 0, -1) x (-1, 0, 0)
  line L0 (0, 15) -> (0, 0) projected
  line L1 (0, 15) -> (-33.4, 15) projected
  line L2 (-33.4, 0) -> (-33.4, 15) projected
  line L3 (-9.5943, 0) -> (-33.4, 0) projected
  line L4 (0, 0) -> (-9.5943, 0) projected
  line L5 (-10.5797, 0) -> (-10.5797, -6.1029) projected
  line L6 (-10.5797, 0) -> (-10.5797, 0.2)
  line L7 (-10.5797, 0.2) -> (-33.4, 0.2)
  point P0 (-31.2, -10.1129)
  dimension "d13" = 0.2
  constraints: 4 end point, 1 perpendicular, 1 point on line, 1 vertical
  measures "d13" distance of L5.start L6.end
extrude "擠出4" cut sketch "草圖4" against normal blind 33.4 contours L7 L6 L3 L2
sketch "草圖5" plane through (2.2, 4.01, 0) normal (1, 0, 0) x (0, 0, -1)
  line L0 (0.0728, 6.3029) -> (12.4596, 6.3029) projected
  line L1 (12.4596, 6.3029) -> (12.4596, 21.1029) projected
  line L2 (12.4596, 21.1029) -> (5.4596, 21.1029) projected
  line L3 (5.4596, 21.1029) -> (0.0728, 6.3029) projected
  point P0 (0, -4.01)
extrude "擠出5" add sketch "草圖5" along normal blind 1
sketch "草圖6" plane through (-31.2, 4.01, -50) normal (-1, 0, 0) x (0, 0, 1)
  line L0 (0, 6.1029) -> (0, 0) projected
  line L1 (50, 0) -> (0, 0) projected
  line L2 (50, 6.1029) -> (50, 0) projected
  line L3 (50, 6.1029) -> (44.5404, 21.1029) projected
  line L4 (44.5404, 21.1029) -> (37.5404, 21.1029) projected
  line L5 (37.5404, 21.1029) -> (37.5404, 6.1029) projected
  line L6 (37.5404, 6.1029) -> (0, 6.1029) projected
  line L7 (37.5404, 21.1029) -> (37.5404, 38.6339)
  line L8 (44.5404, 21.1029) -> (38.1224, 38.7365)
  arc A0 (38.1224, 38.7365) -> (37.5404, 38.6339) centre (37.8404, 38.6339) ccw
  point P0 (50, -4.01)
  dimension "d18" = 0.3
  constraints: 4 end point, 2 point on circle, 2 tangent, 1 centre point, 1 vertical
  measures "d18" radius of A0
extrude "擠出6" add sketch "草圖6" against normal up to surface (34.4 mm away) contours L7 A0 L8 L4
